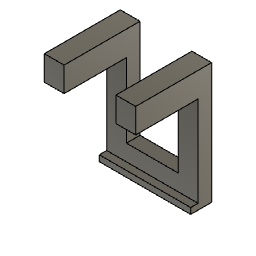
Rack Wedge (Autodesk Fusion 360 design; units mm, degrees)
Autodesk Fusion 360 part; units mm, degrees
sketch "Sketch1" plane through (0, 0, 0) normal (0, 0, 1) x (1, 0, 0)
  line L0 (0, 0) -> (37, 0)
  line L1 (37, 0) -> (37, -5.5)
  line L2 (37, -5.5) -> (0, -5.5)
  line L3 (0, -5.5) -> (0, 0)
  line L4 (0, 0) -> (8, 0)
  line L5 (8, 0) -> (8, -5.5)
  line L6 (8, -5.5) -> (0, -5.5)
  line L7 (0, -5.5) -> (0, 0)
  line L8 (37, 0) -> (29, 0)
  line L9 (29, 0) -> (29, -5.5)
  line L10 (29, -5.5) -> (37, -5.5)
  line L11 (37, -5.5) -> (37, 0)
  dimension "d7" = 37
  dimension "d8" = 5.5
  dimension "d50" = 5.5
  dimension "d51" = 8
  dimension "d52" = 8
  dimension "d53" = 5.5
  constraint horizontal L0
  constraint vertical L1
  constraint horizontal L2
  constraint vertical L3
  constraint coincident L0.start L3.end
  constraint horizontal L4
  constraint vertical L5
  constraint horizontal L6
  constraint vertical L7
  constraint horizontal L8
  constraint vertical L9
  constraint horizontal L10
  constraint vertical L11
  measures "d7" distance of L0.start L0.end
  measures "d8" distance of L0.start L2.end
  measures "d50" distance of L0.start L2.end
  measures "d51" distance of L0.start L4.end
  measures "d52" distance of L0.end L8.end
  measures "d53" distance of L0.end L1.end
extrude "Extrude7" add sketch "Sketch1" along normal blind 49 contours L0 L2 L3 L4 L5 L6 L7 | L0 L1 L2 L8 L9 L10 L11 makes body 1 at (2.6667, 0, 16.3333) makes body 2 at (31.6667, 0, 16.3333)
extrude "Extrude6" add sketch "Sketch1" along normal blind 9 separate body makes body 3
sketch "Sketch6" plane through (0, -5.5, 0) normal (0, -1, 0) x (1, 0, 0)
  line L0 (0, 0) -> (8, 0)
  line L1 (8, 0) -> (8, 49)
  line L2 (8, 49) -> (0, 49)
  line L3 (0, 49) -> (0, 0)
  line L4 (0, 49) -> (8, 49)
  line L5 (8, 49) -> (8, 39)
  line L6 (8, 39) -> (0, 39)
  line L7 (0, 39) -> (0, 49)
  line L8 (29, 49) -> (37, 49)
  line L9 (37, 49) -> (37, 39)
  line L10 (37, 39) -> (29, 39)
  line L11 (29, 39) -> (29, 49)
  line L12 (29, 49) -> (37, 49)
  dimension "d59" = 10
  dimension "d60" = 8
  dimension "d61" = 8
  dimension "d62" = 10
  dimension "d66" = 0
  constraint horizontal L4
  constraint vertical L5
  constraint horizontal L6
  constraint vertical L7
  constraint coincident L2.end L3.start
  constraint horizontal L8
  constraint vertical L9
  constraint horizontal L10
  constraint vertical L11
  measures "d59" distance of L2.end L6.end
  measures "d60" distance of L2.end L1.end
  measures "d61" distance of L8.start L8.end
  measures "d62" distance of L8.start L10.end
  measures "d66" distance of L8 L12
extrude "Extrude8" add sketch "Sketch6" along normal blind 25.25 contours L1 L2 L3 L4 L5 L6 L7 | L8 L9 L10 L11 L12 bodies 1 2 3
sketch "Sketch7" plane through (0, -5.5, 0) normal (0, -1, 0) x (1, 0, 0)
  line L0 (0, 0) -> (37, 0)
  line L1 (37, 0) -> (37, 9)
  line L2 (37, 9) -> (0, 9)
  line L3 (0, 9) -> (0, 0)
  line L4 (0, 0) -> (37, 0)
  line L5 (37, 0) -> (37, 2.4139)
  line L6 (37, 2.4139) -> (0, 2.4139)
  line L7 (0, 2.4139) -> (0, 0)
  dimension "d67" = 37
  dimension "d68" = 2.4139
  constraint horizontal L4
  constraint vertical L5
  constraint horizontal L6
  constraint vertical L7
  constraint coincident L0.start L3.end
  measures "d67" distance of L0.start L0.end
  measures "d68" distance of L0.start L6.end
extrude "Extrude9" add sketch "Sketch7" along normal blind 3 contours L0 L1 L3 L4 L5 L6 L7 bodies 1 2 3
equation "vertical_leg_width = 5.5 mm"
equation "vertical_leg_length = 8 mm"
equation "roof_length = 37 mm"
equation "d7 = roof_length"
equation "d8 = roof_width"
equation "roof_width = 5.5 mm"
equation "roof_thickness = 9 mm"
equation "d47 = roof_thickness"
equation "vertical_leg_height = 40 mm + roof_thickness"
equation "d50 = vertical_leg_width"
equation "d51 = vertical_leg_length"
equation "d52 = vertical_leg_length"
equation "d53 = vertical_leg_width"
equation "d54 = vertical_leg_height"
equation "horizontal_leg_length = 30.75 mm - vertical_leg_width"
equation "horizontal_leg_width = vertical_leg_length"
equation "horizontal_leg_height = 10 mm"
equation "d59 = horizontal_leg_height"
equation "d60 = horizontal_leg_width"
equation "d61 = horizontal_leg_width"
equation "d62 = horizontal_leg_height"
equation "d63 = horizontal_leg_length"
equation "dent_height = 3 mm"
equation "d67 = roof_length"
equation "dent_extrusion = 3 mm"
equation "d70 = dent_extrusion"
